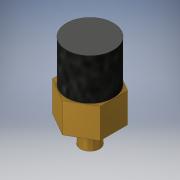
# Autodesk Inventor part: am-2006
Saved by Autodesk Inventor 2016 SP2 (Build 200236200, 236)
## iProperties
Created: 2017-03-28
Part Number: am-2006
Material: Brass
Document SubType Name: Modeling
Designer: smiku
Mass: 173.729 g
Surface Area: 56.9113 cm^2
Volume: 20.4628 cm^3
Density: 8.49 g/cm^3
Appearance: Brass - Polished
Author: smiku
Autodesk Inventor part; units mm, degrees
ref_plane "YZ Plane" through (0, 0, 0) normal (1, 0, 0) x (0, 1, 0)
ref_plane "XZ Plane" through (0, 0, 0) normal (0, 1, 0) x (-1, 0, 0)
ref_plane "XY Plane" through (0, 0, 0) normal (0, 0, 1) x (1, 0, 0)
sketch "Sketch1" plane through (0, 0, 0) normal (0, 1, 0) x (-1, 0, 0)
  circle A0 centre (0, 0) radius 12.7 construction
  line L0 (12.7, -7.3323) -> (0, -14.6647)
  line L1 (0, -14.6647) -> (-12.7, -7.3323)
  line L2 (-12.7, -7.3323) -> (-12.7, 7.3323)
  line L3 (-12.7, 7.3323) -> (0, 14.6647)
  line L4 (0, 14.6647) -> (12.7, 7.3323)
  line L5 (12.7, 7.3323) -> (12.7, -7.3323)
  point P0 (12.7, 0)
  dimension "d0" = 25.4
  constraints: 12 end point, 2 coincident, 1 horizontal alignment, 1 midpoint, 1 vertical, 15 other
extrude "Extrusion1" add sketch "Sketch1" against normal blind 15.875
sketch "Sketch2" plane through (0, -15.875, 0) normal (0, -1, 0) x (1, 0, 0)
  circle A0 centre (0, 0) radius 1.5875
  circle A1 centre (0, 0) radius 5.08
  dimension "d3" = 3.175
  dimension "d4" = 10.16
  constraints: 2 centre point, 2 coincident
  measures "d3" diameter of A0
  measures "d4" diameter of A1
extrude "Extrusion2" add sketch "Sketch2" along normal blind 11.303
sketch "Sketch3" plane through (0, 0, 0) normal (0, 1, 0) x (1, 0, 0)
  circle A0 centre (0, 0) radius 12.446
  dimension "d7" = 24.892
  constraints: 1 centre point, 1 coincident
  measures "d7" diameter of A0
extrude "Extrusion3" add sketch "Sketch3" along normal blind 22.1234 separate body
body "Solid1"
body "Solid2"
